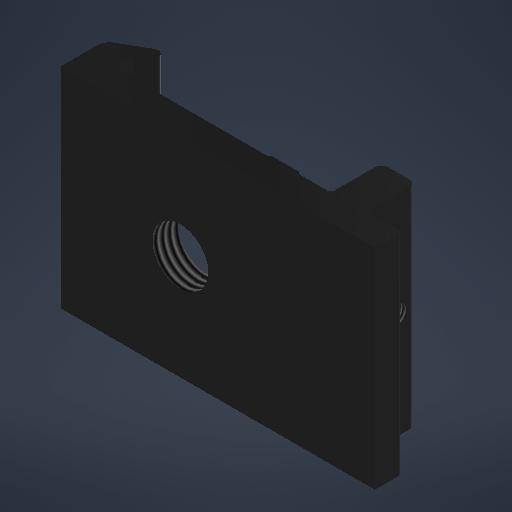
# Autodesk Inventor part: caria_base
Saved by Autodesk Inventor 2026 (Build 300175050, 175E)
## iProperties
Created: 2025-07-09
Part Number: caria_base
Material: UHMW、黒
Document SubType Name: Modeling
Designer: jin20
Density: 0.94 g/cm^3
Appearance: 滑らか - 黒
Author: jin20
Autodesk Inventor part; units mm, degrees
ref_plane "YZ Plane" through (0, 0, 0) normal (1, 0, 0) x (0, 1, 0)
ref_plane "XZ Plane" through (0, 0, 0) normal (0, 1, 0) x (-1, 0, 0)
ref_plane "XY Plane" through (0, 0, 0) normal (0, 0, 1) x (1, 0, 0)
sketch "スケッチ1" plane through (0, 0, 0) normal (0, 1, 0) x (-1, 0, 0)
  line L0 (-49.8489, 61.5411) -> (-49.8489, 83.4411)
  line L1 (-49.8489, 83.4411) -> (10.1511, 83.4411)
  line L2 (10.1511, 83.4411) -> (10.1511, 61.5411)
  line L3 (10.1511, 61.5411) -> (-8.8489, 61.5411)
  line L4 (-8.8489, 56.3412) -> (-8.8489, 74.3411)
  line L5 (-8.8489, 74.3411) -> (-15.9758, 74.3411)
  line L6 (-23.7218, 74.3411) -> (-30.8489, 74.3411)
  line L7 (-30.8489, 74.3411) -> (-30.8489, 56.3412)
  line L8 (-30.8489, 56.3411) -> (-8.8489, 56.3411)
  circle A0 centre (-19.8489, 67.3411) radius 8
  circle A1 centre (-19.8489, 67.3411) radius 7.5
  line L9 (-30.8489, 61.5411) -> (-49.8489, 61.5411)
  line L10 (-49.8489, 75.5411) -> (10.1511, 75.5411)
  line L11 (53.2984, 117.706) -> (53.2984, 177.706)
  line L12 (53.2984, 177.706) -> (143.2984, 177.706)
  line L13 (143.2984, 177.706) -> (143.2984, 117.706)
  line L14 (143.2984, 117.706) -> (53.2984, 117.706)
  circle A2 centre (83.9984, 122.706) radius 1.5
  circle A3 centre (83.9984, 147.706) radius 1.5
  circle A4 centre (93.9984, 147.706) radius 2.25
  circle A5 centre (83.9984, 172.706) radius 1.5
  circle A6 centre (108.9984, 172.706) radius 1.5
  circle A7 centre (133.9984, 172.706) radius 1.5
  circle A8 centre (133.9984, 147.706) radius 1.5
  circle A9 centre (123.9984, 147.706) radius 2.25
  circle A10 centre (108.9984, 147.706) radius 7.5
  circle A11 centre (108.9984, 122.706) radius 1.5
  circle A12 centre (133.9984, 122.706) radius 1.5
  line L15 (174.3262, 83.4411) -> (174.3262, 61.5411)
  line L16 (174.3262, 61.5411) -> (193.3262, 61.5411)
  line L17 (193.3262, 65.4411) -> (193.3262, 56.3412)
  line L18 (193.3262, 56.3411) -> (215.3262, 56.3411)
  line L19 (215.3262, 56.3412) -> (215.3262, 65.4411)
  line L20 (215.3262, 61.5411) -> (234.3263, 61.5411)
  line L21 (234.3263, 61.5411) -> (234.3263, 83.4411)
  line L22 (234.3263, 83.4411) -> (174.3262, 83.4411)
  line L23 (234.3263, 65.4411) -> (174.3262, 65.4411)
  line L24 (143.2984, 25.0403) -> (53.2984, 25.0403)
  line L25 (53.2984, 25.0403) -> (53.2984, -34.9597)
  line L26 (53.2984, -34.9597) -> (143.2984, -34.9597)
  line L27 (143.2984, -34.9597) -> (143.2984, 25.0403)
  line L28 (131.5644, 25.0403) -> (131.5644, -34.9597)
  circle A13 centre (108.9984, -29.9597) radius 1.5
  circle A14 centre (108.9984, -4.9597) radius 7.5
  circle A15 centre (123.9984, -4.9597) radius 2.25
  circle A16 centre (123.9984, -4.9597) radius 4
  circle A17 centre (108.9984, 20.0403) radius 1.5
  circle A18 centre (83.9984, 20.0403) radius 1.5
  line L29 (73.2984, 25.0403) -> (73.2984, 6.0403)
  line L30 (86.3001, -15.9597) -> (86.3001, 6.0403)
  line L31 (86.3001, 6.0403) -> (53.3001, 6.0403)
  line L32 (53.3001, 6.0403) -> (53.3001, -15.9597)
  line L33 (53.3001, -15.9597) -> (86.3001, -15.9597)
  line L34 (73.2984, -15.9597) -> (73.2984, -34.9597)
  line L35 (63.2984, -34.9597) -> (63.2984, -15.9597)
  line L36 (63.2984, 6.0403) -> (63.2984, 25.0403)
  circle A19 centre (83.9984, -29.9597) radius 1.5
  circle A20 centre (93.9984, -4.9597) radius 2.25
  circle A21 centre (93.9984, -4.9597) radius 4
  line L37 (-19.8489, 49.2711) -> (-19.8489, 87.2696)
  line L38 (-6.1616, 67.3411) -> (-35.9585, 67.3411)
  line L39 (83.9984, 23.5784) -> (83.9984, 16.5836)
  circle A22 centre (83.9984, 20.0403) radius 2
  line L40 (80.6576, 20.0403) -> (87.5893, 20.0403)
  line L41 (93.9984, 1.0394) -> (93.9984, -10.6526)
  line L42 (83.9984, -26.503) -> (83.9984, -33.4978)
  circle A23 centre (83.9984, -29.9597) radius 2
  line L43 (80.6576, -29.9597) -> (87.5893, -29.9597)
  line L44 (29.8273, -4.9597) -> (148.6488, -4.9597)
  line L45 (123.9984, -10.6526) -> (123.9984, 1.0394)
  line L46 (112.4368, 20.0403) -> (105.6741, 20.0403)
  circle A24 centre (108.9984, 20.0403) radius 2
  line L47 (108.9984, 32.4142) -> (108.9984, -41.5197)
  circle A25 centre (108.9984, -29.9597) radius 2
  line L48 (105.4074, -29.9597) -> (112.8092, -29.9597)
  circle A26 centre (108.9984, -4.9597) radius 8
  line L49 (108.9984, 111.8823) -> (108.9984, 183.8068)
  circle A27 centre (108.9984, 172.706) radius 2
  line L50 (105.6741, 172.706) -> (112.4368, 172.706)
  line L51 (130.4749, 172.706) -> (137.3391, 172.706)
  circle A28 centre (133.9984, 172.706) radius 2
  line L52 (133.9984, 169.2493) -> (133.9984, 176.2441)
  line L53 (123.9984, 153.3988) -> (123.9984, 141.7069)
  circle A29 centre (123.9984, 147.706) radius 4
  circle A30 centre (133.9984, 147.706) radius 2
  line L54 (133.9984, 151.0572) -> (133.9984, 144.2493)
  line L55 (148.6488, 147.706) -> (29.8273, 147.706)
  circle A31 centre (83.9984, 147.706) radius 2
  line L56 (83.9984, 151.0572) -> (83.9984, 144.2493)
  line L57 (93.9984, 141.7069) -> (93.9984, 153.3988)
  circle A32 centre (93.9984, 147.706) radius 4
  line L58 (83.9984, 169.2493) -> (83.9984, 176.2441)
  circle A33 centre (83.9984, 172.706) radius 2
  line L59 (80.6576, 172.706) -> (87.5893, 172.706)
  circle A34 centre (108.9984, 147.706) radius 8
  circle A35 centre (108.9984, 122.706) radius 2
  line L60 (105.4074, 122.706) -> (112.8092, 122.706)
  line L61 (130.8446, 122.706) -> (137.3391, 122.706)
  circle A36 centre (133.9984, 122.706) radius 2
  line L62 (133.9984, 126.1627) -> (133.9984, 119.1679)
  line L63 (87.5893, 122.706) -> (80.6576, 122.706)
  circle A37 centre (83.9984, 122.706) radius 2
  line L64 (83.9984, 126.1627) -> (83.9984, 119.1679)
  line L65 (204.3262, 87.2696) -> (204.3262, 49.2711)
  line L66 (176.3262, 70.0686) -> (232.3263, 70.0686)
  line L67 (82.1365, 4.0403) -> (82.1365, -13.9597)
  line L68 (51.8001, 144.706) -> (51.8001, 150.706)
  line L69 (53.2984, 150.706) -> (51.8001, 150.706)
  line L70 (53.2984, 144.706) -> (51.8001, 144.706)
  line L71 (33.8001, 155.206) -> (33.8001, 140.206)
  line L72 (33.8001, 140.206) -> (34.3001, 139.706)
  line L73 (34.3001, 139.706) -> (51.3001, 139.706)
  line L74 (51.3001, 139.706) -> (51.8001, 140.206)
  line L75 (51.8001, 140.206) -> (51.8001, 155.206)
  line L76 (51.8001, 155.206) -> (51.3001, 155.706)
  line L77 (51.3001, 155.706) -> (34.3001, 155.706)
  line L78 (34.3001, 155.706) -> (33.8001, 155.206)
  line L79 (34.3001, 155.706) -> (34.3001, 139.706)
  line L80 (51.3001, 139.706) -> (51.3001, 155.706)
  line L81 (51.8001, -7.9597) -> (51.8001, -1.9597)
  line L82 (53.3001, -1.9597) -> (51.8001, -1.9597)
  line L83 (53.3001, -7.9597) -> (51.8001, -7.9597)
  line L84 (33.8001, 2.5403) -> (33.8001, -12.4597)
  line L85 (33.8001, -12.4597) -> (34.3001, -12.9597)
  line L86 (34.3001, -12.9597) -> (51.3001, -12.9597)
  line L87 (51.3001, -12.9597) -> (51.8001, -12.4597)
  line L88 (51.8001, -12.4597) -> (51.8001, 2.5403)
  line L89 (51.8001, 2.5403) -> (51.3001, 3.0403)
  line L90 (51.3001, 3.0403) -> (34.3001, 3.0403)
  line L91 (34.3001, 3.0403) -> (33.8001, 2.5403)
  line L92 (34.3001, 3.0403) -> (34.3001, -12.9597)
  line L93 (51.3001, -12.9597) -> (51.3001, 3.0403)
  line L94 (28.0972, 67.3411) -> (83.3407, 67.3411)
  line L95 (82.8984, 75.4411) -> (90.6984, 75.4411)
  line L96 (127.3984, 75.4411) -> (133.1984, 75.4411)
  line L97 (134.7552, 70.5411) -> (131.5724, 67.3583)
  line L98 (82.4415, 71.3411) -> (86.3001, 67.4825)
  line L99 (78.3001, 69.4911) -> (75.8001, 69.4911)
  line L100 (78.3001, 65.1911) -> (75.8001, 65.1911)
  line L101 (75.8001, 64.8411) -> (75.8001, 69.8411)
  line L102 (75.3001, 70.3411) -> (73.1569, 70.3411)
  line L103 (75.3001, 64.3411) -> (73.1569, 64.3411)
  line L104 (75.8001, 69.8411) -> (73.1569, 69.8411)
  line L105 (75.8001, 64.8411) -> (73.1569, 64.8411)
  line L106 (51.8001, 64.3411) -> (51.8001, 70.3411)
  line L107 (53.3001, 70.3411) -> (51.8001, 70.3411)
  line L108 (53.3001, 64.3411) -> (51.8001, 64.3411)
  line L109 (33.8001, 74.8411) -> (33.8001, 59.8411)
  line L110 (33.8001, 59.8411) -> (34.3001, 59.3411)
  line L111 (34.3001, 59.3411) -> (51.3001, 59.3411)
  line L112 (51.3001, 59.3411) -> (51.8001, 59.8411)
  line L113 (51.8001, 59.8411) -> (51.8001, 74.8411)
  line L114 (51.8001, 74.8411) -> (51.3001, 75.3411)
  line L115 (51.3001, 75.3411) -> (34.3001, 75.3411)
  line L116 (34.3001, 75.3411) -> (33.8001, 74.8411)
  line L117 (34.3001, 75.3411) -> (34.3001, 59.3411)
  line L118 (51.3001, 59.3411) -> (51.3001, 75.3411)
  line L119 (54.3001, 74.3411) -> (60.3001, 74.3411)
  line L120 (54.3001, 56.3411) -> (80.2082, 56.3411)
  line L121 (53.3001, 57.3411) -> (53.3001, 73.3411)
  line L122 (86.3001, 60.5366) -> (86.3001, 67.4825)
  line L123 (61.3001, 62.3411) -> (61.3001, 73.3411)
  line L124 (62.3001, 61.3411) -> (77.3001, 61.3411)
  line L125 (78.3001, 62.3411) -> (78.3001, 70.3411)
  line L126 (79.3001, 71.3411) -> (82.4415, 71.3411)
  line L127 (82.1365, 57.0429) -> (86.3001, 60.5366)
  arc A38 (80.2082, 56.3411) -> (82.1365, 57.0429) centre (80.2082, 59.3411) ccw
  arc A39 (54.3001, 74.3411) -> (53.3001, 73.3411) centre (54.3001, 73.3411) ccw
  arc A40 (61.3001, 73.3411) -> (60.3001, 74.3411) centre (60.3001, 73.3411) ccw
  arc A41 (53.3001, 57.3411) -> (54.3001, 56.3411) centre (54.3001, 57.3411) ccw
  arc A42 (61.3001, 62.3411) -> (62.3001, 61.3411) centre (62.3001, 62.3411) ccw
  arc A43 (77.3001, 61.3411) -> (78.3001, 62.3411) centre (77.3001, 62.3411) ccw
  arc A44 (79.3001, 71.3411) -> (78.3001, 70.3411) centre (79.3001, 70.3411) ccw
  line L128 (63.1569, 70.3411) -> (61.3001, 70.3411)
  line L129 (63.1569, 69.8411) -> (61.3001, 69.8411)
  line L130 (63.1569, 64.8411) -> (61.3001, 64.8411)
  line L131 (63.1569, 64.3411) -> (61.3001, 64.3411)
  line L132 (75.3001, 70.3411) -> (75.8001, 69.8411)
  line L133 (75.3001, 64.3411) -> (75.8001, 64.8411)
  arc A45 (63.2984, 63.5411) -> (65.2984, 61.5411) centre (65.2984, 63.5411) ccw
  line L134 (65.2984, 61.5411) -> (71.2984, 61.5411)
  arc A46 (71.2984, 61.5411) -> (73.2984, 63.5411) centre (71.2984, 63.5411) ccw
  line L135 (73.2984, 63.5411) -> (73.2984, 75.0411)
  line L136 (135.2984, 75.8411) -> (135.2984, 70.7411)
  line L137 (143.2984, 72.6666) -> (143.2984, 83.4411)
  line L138 (143.2984, 83.4411) -> (53.2984, 83.4411)
  line L139 (53.2984, 83.4411) -> (53.2984, 76.5411)
  arc A47 (53.2984, 76.5411) -> (54.2984, 75.5411) centre (54.2984, 76.5411) ccw
  line L140 (54.2984, 75.5411) -> (62.2984, 75.5411)
  arc A48 (63.2984, 74.5411) -> (62.2984, 75.5411) centre (62.2984, 74.5411) ccw
  line L141 (63.2984, 74.5411) -> (63.2984, 63.5411)
  line L142 (74.2984, 76.0411) -> (82.2984, 76.0411)
  line L143 (133.7984, 76.0411) -> (133.1984, 75.4411)
  line L144 (127.3984, 75.4411) -> (126.7984, 76.0411)
  line L145 (90.6984, 75.4411) -> (91.2984, 76.0411)
  line L146 (82.8984, 75.4411) -> (82.2984, 76.0411)
  line L147 (91.2984, 76.0411) -> (126.7984, 76.0411)
  arc A49 (74.2984, 76.0411) -> (73.2984, 75.0411) centre (74.2984, 75.0411) ccw
  line L148 (133.7984, 76.0411) -> (135.0984, 76.0411)
  arc A50 (135.2984, 75.8411) -> (135.0984, 76.0411) centre (135.0984, 75.8411) ccw
  line L149 (135.0984, 70.5411) -> (134.7552, 70.5411)
  arc A51 (135.0984, 70.5411) -> (135.2984, 70.7411) centre (135.0984, 70.7411) ccw
  arc A52 (131.5724, 67.3583) -> (134.1894, 65.6755) centre (133.3144, 67.1911) ccw
  line L150 (134.1894, 65.6755) -> (141.7984, 70.0686)
  arc A53 (141.7984, 70.0686) -> (143.2984, 72.6666) centre (140.2984, 72.6666) ccw
  line L151 (124.9984, 127.8911) -> (124.9984, 123.5209)
  line L152 (127.1835, 125.706) -> (122.8133, 125.706)
  circle A54 centre (124.9984, 125.706) radius 1
  circle A55 centre (124.9984, 125.706) radius 1.5
  line L153 (124.9984, 167.5209) -> (124.9984, 171.8911)
  line L154 (127.1835, 169.706) -> (122.8133, 169.706)
  circle A56 centre (124.9984, 169.706) radius 1
  circle A57 centre (124.9984, 169.706) radius 1.5
  line L155 (58.9984, 127.8911) -> (58.9984, 123.5209)
  line L156 (61.1835, 125.706) -> (56.8133, 125.706)
  circle A58 centre (58.9984, 125.706) radius 1
  circle A59 centre (58.9984, 125.706) radius 1.5
  line L157 (58.9984, 167.5209) -> (58.9984, 171.8911)
  line L158 (61.1835, 169.706) -> (56.8133, 169.706)
  circle A60 centre (58.9984, 169.706) radius 1
  circle A61 centre (58.9984, 169.706) radius 1.5
  line L159 (34.3001, 154.706) -> (49.1751, 154.706)
  line L160 (34.3001, 153.706) -> (47.0501, 153.706)
  line L161 (34.3001, 152.706) -> (44.9251, 152.706)
  line L162 (34.3001, 151.706) -> (42.8001, 151.706)
  line L163 (34.3001, 150.706) -> (40.6751, 150.706)
  line L164 (34.3001, 149.706) -> (38.5501, 149.706)
  line L165 (34.3001, 148.706) -> (36.4251, 148.706)
  line L166 (34.3001, 2.0403) -> (49.1751, 2.0403)
  line L167 (34.3001, 1.0403) -> (47.0501, 1.0403)
  line L168 (34.3001, 0.0403) -> (44.9251, 0.0403)
  line L169 (34.3001, -0.9597) -> (42.8001, -0.9597)
  line L170 (34.3001, -1.9597) -> (40.6751, -1.9597)
  line L171 (34.3001, -2.9597) -> (38.5501, -2.9597)
  line L172 (34.3001, -3.9597) -> (36.4251, -3.9597)
  line L173 (108.9984, 51.8579) -> (108.9984, 88.7279)
  line L174 (34.3001, 74.3411) -> (49.1751, 74.3411)
  line L175 (34.3001, 73.3411) -> (47.0501, 73.3411)
  line L176 (34.3001, 72.3411) -> (44.9251, 72.3411)
  line L177 (34.3001, 71.3411) -> (42.8001, 71.3411)
  line L178 (34.3001, 70.3411) -> (40.6751, 70.3411)
  line L179 (34.3001, 69.3411) -> (38.5501, 69.3411)
  line L180 (34.3001, 68.3411) -> (36.4251, 68.3411)
  point P0 (0, 0)
  point P1 (209.8216, -24.5126)
  point P2 (209.8216, -11.7034)
  point P3 (131.5724, 67.3583)
  point P4 (134.1894, 65.6755)
  point P5 (141.7984, 70.0686)
  point P6 (54.2984, 75.5411)
  point P7 (63.2984, 67.3411)
  point P8 (73.2984, 67.3411)
  constraints: 362 end point, 62 centre point, 32 point on circle, 2 other
extrude "押し出し1" add sketch "スケッチ1" along normal blind 60 contours L141 A48 L140 A47 L139 L138 L173 L147 L145 L95 L146 L142 A49 L135 L94 | L94 L135 A46 L134 A45 L141 | L138 L137 A53 L150 A52 L97 L149 A51 L136 A50 L148 L143 L96 L144 L147 L173
sketch "スケッチ2" plane through (-143.2984, 0, 83.4411) normal (0, 0, 1) x (1, 0, 0)
  line L0 (0, 0) -> (0, 60) projected
  line L1 (0, 30) -> (34.3, 30) construction
  circle A0 centre (34.3, 30) radius 8
  point P0 (143.2984, 0)
  dimension "d2" = 34.3
  dimension "d3" = 16
  constraints: 2 end point, 1 centre point, 1 coincident, 1 horizontal, 1 midpoint
  measures "d2" distance of L1.start L1.end
  measures "d3" diameter of A0
extrude "押し出し2" cut sketch "スケッチ2" against normal through all
thread "ねじ1" size "M16x2" class "6H" standard "ANSI Metric M Profile" full length
sketch "スケッチ4" plane through (-63.2984, 0, 74.5411) normal (1, 0, 0) x (0, 0, -1)
  line L0 (13, 0) -> (13, 60) projected
  line L1 (13, 30) -> (7.2, 30) construction
  circle A0 centre (7.2, 30) radius 3
  point P0 (74.5411, 0)
  dimension "d14" = 5.8
  dimension "d15" = 6
  constraints: 2 end point, 1 centre point, 1 coincident, 1 horizontal, 1 midpoint
  measures "d14" distance of L1.start L1.end
  measures "d15" diameter of A0
extrude "押し出し4" cut sketch "スケッチ4" against normal blind 10
thread "ねじ3" size "M6x1" class "6H" standard "ANSI Metric M Profile" full length
